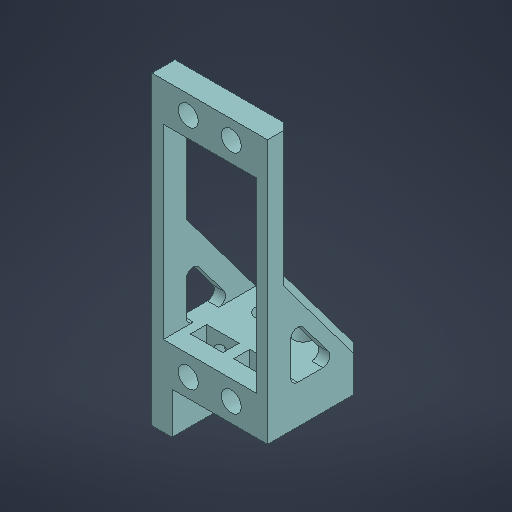
# Autodesk Inventor part: BIGServoHolder
Saved by Autodesk Inventor 2025.1 (Build 291241000, 241)
## iProperties
Created: 2025-02-24
Part Number: BIGServoHolder
Material: Generic
Document SubType Name: Modeling
Designer: 13156
Density: 1 g/cm^3
Appearance: Default
Author: 13156
## iProperties of the stored document BIGServoHolder_3DPrint.ipt
Created: 2025-03-04
Part Number: BIGServoHolder_3DPrint
Material: Generic
Document SubType Name: Modeling
Designer: jerem
Density: 1 g/cm^3
Appearance: Default
Author: jerem
Autodesk Inventor part; units mm, degrees
ref_plane "YZ Plane" through (0, 0, 0) normal (1, 0, 0) x (0, 1, 0)
ref_plane "XZ Plane" through (0, 0, 0) normal (0, 1, 0) x (-1, 0, 0)
sketch "Sketch1" plane through (0, 0, 0) normal (0, 0, 1) x (1, 0, 0)
  line L0 (-12.5, 28.5) -> (12.5, 28.5)
  line L1 (12.5, 28.5) -> (12.5, -28.5)
  line L2 (12.5, -28.5) -> (-12.5, -28.5)
  line L3 (-12.5, -28.5) -> (-12.5, 28.5)
  line L4 (-10.05, 20.15) -> (10.05, 20.15)
  line L5 (10.05, 20.15) -> (10.05, -20.15)
  line L6 (10.05, -20.15) -> (-10.05, -20.15)
  line L7 (-10.05, -20.15) -> (-10.05, 20.15)
  line L8 (0, 0) -> (0, 17.7516) construction
  line L9 (0, 0) -> (17.0454, 0) construction
  line L10 (-12.5, -28.5) -> (12.5, -28.5)
  line L11 (12.5, -28.5) -> (12.5, -20.15)
  line L12 (12.5, -20.15) -> (-12.5, -20.15)
  line L13 (-12.5, -20.15) -> (-12.5, -28.5)
  circle A0 centre (-4.65, 24.5) radius 2.175
  circle A1 centre (4.65, 24.475) radius 2.175
  circle A2 centre (-4.6492, -24.5) radius 2.175
  circle A3 centre (4.65, -24.375) radius 2.175
  point P0 (12.5, -24.325)
  dimension "d0" = 40.3
  dimension "d1" = 20.1
  dimension "d2" = 57
  dimension "d3" = 25
  dimension "d4" = 4.35
  dimension "d5" = 4.325
  dimension "d6" = 4.35
  dimension "d8" = 4.35
  dimension "d9" = 5.4
  dimension "d13" = 5.4
  dimension "d28" = 48.85
  dimension "d29" = 9.3
  dimension "d30" = 9.3
  constraints: 28 end point, 6 parallel, 4 centre point, 4 horizontal, 3 equal radius, 3 perpendicular, 1 collinear, 1 midpoint, 1 point on line, 1 vertical, 4 other
  measures "d0" distance between parallel lines of L6 L4
  measures "d1" distance between parallel lines of L5 L7
  measures "d2" distance between parallel lines of L2 L0
  measures "d3" distance between parallel lines of L1 L3
  measures "d4" diameter of A1
  measures "d5" distance from line of L4 A1.centre
  measures "d6" distance from line of L4 A0.centre
  measures "d8" distance from line of L6 A2.centre
  measures "d9" distance from line of L5 A1.centre
  measures "d13" distance from line of L5 A3.centre
  measures "d28" distance of A1.centre A3.centre
  measures "d29" distance of A2.centre A3.centre
  measures "d30" distance of A1.centre A0.centre
extrude "Extrusion1" add sketch "Sketch1" along normal blind 5 contours L0 L1 L12 L5 L4 L7 L3 | L12 L6 L1 L2 L3
extrude "Extrusion2" add sketch "Sketch1" against normal blind 15 contours L12 L6 L1 L2 L3 | A2 | A3
extrude "Extrusion3" cut sketch "Sketch1" against normal blind 10 from surface at 5 contours A2 | A3
sketch "Sketch2" plane through (-10.05, -20.15, 5) normal (0, 1, 0) x (1, 0, 0)
  circle A0 centre (5.9, 16) radius 1.1
  circle A1 centre (14.2, 16) radius 1.1
  line L0 (0, 0) -> (20.1, 0) construction
  line L1 (10.05, 0) -> (10.05, 23.167) construction
  line L2 (-2.45, 20) -> (22.55, 20) projected
  circle A2 centre (14.2, 16) radius 2
  circle A3 centre (5.9, 16) radius 2
  point P0 (10.05, 5)
  dimension "d20" = 2.2
  dimension "d21" = 8.3
  dimension "d22" = 4
  dimension "d23" = 4
  constraints: 4 centre point, 2 coincident, 2 end point, 2 equal radius, 1 midpoint, 1 vertical, 1 other
  measures "d20" diameter of A0
  measures "d21" distance of A1.centre A0.centre
  measures "d22" distance from line of L2 A1.centre
  measures "d23" diameter of A2
extrude "Extrusion4" cut sketch "Sketch2" against normal blind 10 contours A0 | A1
extrude "Extrusion5" cut sketch "Sketch2" against normal blind 3 contours A0 | A1 | A2 | A3
sketch "Sketch3" plane through (12.5, -20.15, 0) normal (1, 0, 0) x (0, 0, -1)
  line L0 (0, 48.65) -> (-5, 48.65) construction
  line L1 (-5, 48.65) -> (38.6712, 48.65) construction
  line L2 (0, 0) -> (-5, 0) construction
  line L3 (-5, 0) -> (38.6712, 0) construction
  line L4 (0, 20) -> (15, 0)
  line L5 (0, 20) -> (0, 13.3333)
  line L6 (0, 13.3333) -> (10, 0)
  line L7 (10, 0) -> (15, 0)
  line L8 (15, 0) -> (15, -8.35) construction
  line L9 (15, -0.9137) -> (15, 2.4866) construction
  line L10 (-5, 0) -> (15, 0)
  line L11 (15, 0) -> (15, -17.35)
  line L12 (15, -17.35) -> (-5, -17.35)
  line L13 (-5, -17.35) -> (-5, 0)
  circle A0 centre (5, -13.35) radius 1.25
  line L14 (0, 0) -> (0, 48.65) projected
  line L15 (0, 48.65) -> (0, 0) projected
  line L16 (0, 0) -> (15, 0) projected
  line L17 (15, -8.35) -> (15, 0) projected
  line L18 (15, -8.35) -> (-5, -8.35) projected
  line L19 (-5, 48.65) -> (-5, -8.35) projected
  line L20 (0, 48.65) -> (-5, 48.65) projected
  point P0 (0, 20.15)
  dimension "d31" = 4
  dimension "d39" = 2.5
  dimension "d41" = 10
  dimension "d46" = 5
  dimension "d59" = 9
  dimension "d63" = 20
  constraints: 22 end point, 3 horizontal, 3 parallel, 3 point on line, 2 collinear, 1 centre point, 1 perpendicular, 1 vertical
  measures "d31" distance between parallel lines of L6 L4
  measures "d39" diameter of A0
  measures "d41" distance from line of L11 A0.centre
  measures "d46" distance from line of L18 A0.centre
  measures "d59" distance between parallel lines of L12 L18
  measures "d63" distance of L2.start L4.start
extrude "Extrusion6" add sketch "Sketch3" against normal up to surface (2.45 mm away) contours L4 L7 L6 L5
extrude "Extrusion7" add sketch "Sketch3" along normal blind 4.35 from surface at -25 contours L11 L18 L13 L10 L7 | L11 L12 L13 L18 | A0
extrude "Extrusion8" cut sketch "Sketch3" against normal blind 35.65 contours A0
ref_plane "Work Plane2" through (0, -28.5, 5) normal (1, 0, 0) x (0, 0, -1)
mirror "Mirror1" about plane through (0, -28.5, 5) normal (1, 0, 0) of "Extrusion6"
fillet "Fillet1" radius 1.5 6 edges at (11.275, -20.15, 0) (11.275, -6.8167, 0) (11.275, -20.15, -10) (-11.275, -20.15, -10) (-11.275, -6.8167, 0) (-11.275, -20.15, 0)
chamfer "Chamfer1" distance 1.5 angle 45 3 edges at (12.5, -24.325, -15) (12.5, -10.15, -7.5) (12.5, 14.175, 0)
sketch "Sketch4" plane through (-12.5, 28.5, 0) normal (-1, 0, 0) x (0, 0, 1)
  circle A0 centre (-5, -62) radius 1.25 projected
  circle A1 centre (-5, -62) radius 2
  point P0 (0, -28.5)
  dimension "d51" = 4
  constraints: 1 centre point, 1 coincident
  measures "d51" diameter of A1
extrude "Extrusion9" cut sketch "Sketch4" against normal blind 3
sketch "Sketch5" plane through (-10.05, -20.15, 5) normal (0, 1, 0) x (1, 0, 0)
  line L0 (1.9008, 7.5) -> (8.9008, 7.5)
  line L1 (8.9008, 7.5) -> (8.9008, 4)
  line L2 (8.9008, 4) -> (1.9008, 4)
  line L3 (1.9008, 4) -> (1.9008, 7.5)
  line L4 (11.2, 7.5) -> (18.2, 7.5)
  line L5 (18.2, 7.5) -> (18.2, 4)
  line L6 (18.2, 4) -> (11.2, 4)
  line L7 (11.2, 4) -> (11.2, 7.5)
  line L8 (22.55, 0) -> (-2.45, 0) projected
  line L9 (5.4008, 4) -> (5.4008, 0) construction
  line L10 (14.7, 4) -> (14.7, 0) construction
  line L11 (7.5758, 0) -> (3.2258, 0) construction
  line L12 (16.875, 0) -> (12.525, 0) construction
  dimension "d54" = 7
  dimension "d55" = 3.5
  dimension "d56" = 4
  constraints: 20 end point, 4 midpoint, 4 parallel, 4 perpendicular, 3 equal length, 2 horizontal, 2 point on line
  measures "d54" distance of L1.end L2.end
  measures "d55" distance of L2.end L0.start
  measures "d56" distance of L9.start L9.end
extrude "Extrusion10" cut sketch "Sketch5" against normal blind 10
chamfer "Chamfer2" distance 9 angle 45 1 edges at (-10.325, -37.5, -15)
equation "\"d8\" = d6"
equation "\"d13\" = d9"
body "Solid1"
